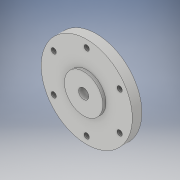
# Autodesk Inventor part: Mecanum Wheel Adapter Plate
Saved by Autodesk Inventor 2017 (Build 210142000, 142)
## iProperties
Created: 2017-07-29
Part Number: Mecanum Wheel Adapter Plate
Material: Generic
Document SubType Name: Modeling
Designer: User
Density: 1 g/cm^3
Appearance: Default
Author: User
Autodesk Inventor part; units mm, degrees
ref_plane "YZ Plane" through (0, 0, 0) normal (1, 0, 0) x (0, 1, 0)
ref_plane "XZ Plane" through (0, 0, 0) normal (0, 1, 0) x (-1, 0, 0)
ref_plane "XY Plane" through (0, 0, 0) normal (0, 0, 1) x (1, 0, 0)
sketch "Sketch1" plane through (0, 0, 0) normal (0, 0, 1) x (1, 0, 0)
  circle A0 centre (0, 0) radius 28.3972
  dimension "d0" = 56.7944
  constraints: 1 centre point, 1 coincident
  measures "d0" diameter of A0
extrude "Extrusion1" add sketch "Sketch1" along normal blind 5.9944
sketch "Sketch2" plane through (0, 0, 5.9944) normal (0, 0, 1) x (1, 0, 0)
  point P0 (0, 0)
  point P1 (0, 0)
  constraints: 1 coincident
hole "Hole1" at (0, 0, 5.9944) direction (0, 0, -1) diameter 6.35 depth 5.9944
sketch "Sketch3" plane through (0, 0, 0) normal (0, 0, -1) x (-1, 0, 0)
  circle A0 centre (0, 0) radius 3.175 construction
  line L0 (0, 0) -> (0, 23.749) construction
  dimension "d10" = 23.749
  constraints: 2 end point, 1 coincident, 1 vertical
  measures "d10" distance of L0.start L0.end
hole "Hole2" at (0, 23.749, 0) direction (0, 0, 1) diameter 3.302 depth 12.2936 tip angle 118 thread size "8-32 UNC" class "2B" standard "ANSI Unified Screw Threads"
pattern_circular "Circular Pattern1" count 6 over 360 about axis through (0, 0, 2.9972) along (0, 0, 1) of "Hole2"
sketch "Sketch4" plane through (0, 0, 5.9944) normal (0, 0, 1) x (1, 0, 0)
  circle A0 centre (0, 0) radius 3.175 projected
  circle A1 centre (0, 0) radius 11.9888
  dimension "d22" = 23.9776
  constraints: 1 centre point, 1 coincident
  measures "d22" diameter of A1
extrude "Extrusion2" add sketch "Sketch4" along normal blind 1.905
body "Solid1"
